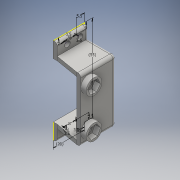
# Autodesk Inventor part: SwitchMount
Saved by Autodesk Inventor 2016 (Build 200138000, 138)
## iProperties
Created: 2026-04-02
Part Number: SwitchMount
Material: Generic
Document SubType Name: Modeling
Designer: Steve
Density: 1 g/cm^3
Appearance: Default
Author: Steve
Autodesk Inventor part; units mm, degrees
ref_plane "YZ Plane" through (0, 0, 0) normal (1, 0, 0) x (0, 1, 0)
ref_plane "XZ Plane" through (0, 0, 0) normal (0, 1, 0) x (-1, 0, 0)
ref_plane "XY Plane" through (0, 0, 0) normal (0, 0, 1) x (1, 0, 0)
sketch "Sketch1" plane through (0, 0, 0) normal (0, 1, 0) x (-1, 0, 0)
  line L0 (10, 17.5) -> (-10, 17.5)
  line L1 (-10, 17.5) -> (-10, -17.5)
  line L2 (-10, -17.5) -> (10, -17.5)
  line L3 (10, -17.5) -> (10, 17.5)
  line L4 (6.5, 5.2) -> (-6.5, 5.2)
  line L5 (-6.5, 5.2) -> (-6.5, -14)
  line L6 (-6.5, -14) -> (6.5, -14)
  line L7 (6.5, -14) -> (6.5, 5.2)
  circle A0 centre (5, 12.5) radius 2.55
  line L8 (7.6, 6.2) -> (-7.6, 6.2)
  line L9 (-7.6, 6.2) -> (-7.6, -15)
  line L10 (-7.6, -15) -> (7.6, -15)
  line L11 (7.6, -15) -> (7.6, 6.2)
  point P0 (0, 0)
  dimension "d0" = 35
  dimension "d1" = 20
  dimension "d2" = 17.5
  dimension "d3" = 10
  dimension "d4" = 19.2
  dimension "d5" = 13
  dimension "d6" = 3.5
  dimension "d7" = 3.5
  dimension "d8" = 5.1
  dimension "d9" = 5
  dimension "d10" = 5
  dimension "d11" = 1.1
  dimension "d12" = 1.1
  dimension "d13" = 15.2
  dimension "d14" = 1
  dimension "d15" = 1
  dimension "d16" = 21.2
  dimension "d42" = 6.3
  constraints: 24 end point, 6 parallel, 3 horizontal, 3 perpendicular, 1 centre point
  measures "d0" distance of L2.end L0.start
  measures "d1" distance of L1.end L2.end
  measures "d2" distance from line of L0 point (0, 0)
  measures "d3" distance from line of L3 point (0, 0)
  measures "d4" distance of L6.end L4.start
  measures "d5" distance of L5.end L6.end
  measures "d6" distance between parallel lines of L3 L7
  measures "d7" distance between parallel lines of L2 L6
  measures "d8" diameter of A0
  measures "d9" distance from line of L3 A0.centre
  measures "d10" distance from line of L0 A0.centre
  measures "d11" distance between parallel lines of L11 L7
  measures "d12" distance between parallel lines of L9 L5
  measures "d13" distance of L9.end L10.end
  measures "d14" distance between parallel lines of L8 L4
  measures "d15" distance between parallel lines of L10 L6
  measures "d16" distance of L10.end L8.start
  measures "d42" distance from line of L8 A0.centre
extrude "Extrusion1" add sketch "Sketch1" along normal blind 2.5 contours L3 L2 L1 L0
extrude "Extrusion2" add sketch "Sketch1" along normal blind 1.5 contours L11 L10 L9 L8
sketch "Sketch2" plane through (-10, 0, -17.5) normal (-1, 0, 0) x (0, 0, 1)
  line L0 (35, 2.5) -> (0, 2.5) projected
  line L1 (0, 2.5) -> (-10, 2.5)
  line L2 (-10, 2.5) -> (-10, -17.5)
  line L3 (-10, -17.5) -> (0, -17.5)
  line L4 (0, -17.5) -> (0, 2.5)
  line L5 (35, 2.5) -> (45, 2.5)
  line L6 (45, 2.5) -> (45, -17.5)
  line L7 (45, -17.5) -> (35, -17.5)
  line L8 (35, -17.5) -> (35, 2.5)
  point P0 (17.5, 0)
  dimension "d21" = 10
  dimension "d22" = 20
  dimension "d23" = 10
  dimension "d24" = 20
  constraints: 16 end point, 4 parallel, 2 horizontal, 2 perpendicular
  measures "d21" distance of L3.end L2.end
  measures "d22" distance of L2.end L1.end
  measures "d23" distance of L6.end L7.end
  measures "d24" distance of L5.end L6.end
extrude "Extrusion3" add sketch "Sketch2" against normal blind 2.5
sketch "Sketch3" plane through (-10, -17.5, -27.5) normal (-1, 0, 0) x (0, 0, 1)
  circle A0 centre (51, 14.5) radius 1.75
  circle A1 centre (4, 14.5) radius 1.75
  circle A2 centre (4, 6.5) radius 1.75
  line L0 (55, 20) -> (0, 20) projected
  line L1 (0, 0) -> (10, 0) projected
  line L2 (55, 0) -> (55, 20) projected
  line L3 (0, 20) -> (0, 0) projected
  circle A3 centre (51, 6.5) radius 1.75
  point P0 (27.5, 17.5)
  dimension "d27" = 3.5
  dimension "d28" = 3.5
  dimension "d29" = 3.5
  dimension "d30" = 5.5
  dimension "d31" = 5.5
  dimension "d32" = 8
  dimension "d34" = 4
  dimension "d35" = 4
  dimension "d36" = 4
  dimension "d83" = 3.5
  dimension "d84" = 4
  dimension "d85" = 8
  dimension "d113" = 20
  dimension "d114" = 55
  constraints: 4 centre point
  measures "d27" diameter of A0
  measures "d28" diameter of A1
  measures "d29" diameter of A2
  measures "d30" distance from line of L0 A0.centre
  measures "d31" distance from line of L0 A1.centre
  measures "d32" distance of A2.centre A1.centre
  measures "d34" distance from line of L2 A0.centre
  measures "d35" distance from line of L3 A1.centre
  measures "d36" distance from line of L3 A2.centre
  measures "d83" diameter of A3
  measures "d84" distance from line of L2 A3.centre
  measures "d85" distance of A0.centre A3.centre
  measures "d113" distance of L0.end L1.start
  measures "d114" distance of L0.start L0.end
sketch "Sketch5" plane through (0, 0, 0) normal (0, -1, 0) x (1, 0, 0)
  line L0 (10, 17.5) -> (10, -17.5) projected
  line L1 (-7.5, 17.5) -> (10, 17.5) projected
  line L2 (10, -17.5) -> (7.5, -17.5)
  line L3 (7.5, -17.5) -> (7.5, 17.5)
  line L4 (7.5, 17.5) -> (10, 17.5)
  line L5 (10, 17.5) -> (10, -17.5)
  point P0 (0, 0)
  dimension "d41" = 2.5
  constraints: 8 end point, 2 parallel, 1 horizontal, 1 perpendicular, 1 point on line
  measures "d41" distance of L3.end L4.end
extrude "Extrusion6" add sketch "Sketch5" along normal blind 20
sketch "Sketch9" plane through (-7.5, 2.5, 17.5) normal (0, 0, 1) x (1, 0, 0)
  line L0 (0, 0) -> (17.5, 0) projected
  line L1 (17.5, -22.5) -> (17.5, 0) projected
  line L2 (17.5, 0) -> (17.5, -22.5)
  line L3 (17.5, -22.5) -> (15, -22.5)
  line L4 (15, -22.5) -> (0, -20)
  line L5 (0, -20) -> (0, 0)
  line L6 (0, 0) -> (17.5, 0)
  point P0 (7.5, -2.5)
  constraints: 10 end point, 1 collinear, 1 parallel, 1 perpendicular, 1 vertical
extrude "Extrusion11" add sketch "Sketch9" along normal blind 2.5
sketch "Sketch11" plane through (10, 2.5, -17.5) normal (0, 0, -1) x (-1, 0, 0)
  line L0 (0, 0) -> (17.5, 0) projected
  line L1 (17.5, 0) -> (0, 0)
  line L2 (0, 0) -> (0, -22.5)
  line L3 (2.5, -22.5) -> (0, -22.5) projected
  line L4 (0, -22.5) -> (2.5, -22.5)
  line L5 (17.5, -20) -> (2.5, -22.5) projected
  line L6 (2.5, -22.5) -> (17.5, -20)
  line L7 (17.5, -20) -> (17.5, 0)
  point P0 (10, -2.5)
  constraints: 10 end point, 2 collinear, 1 horizontal, 1 parallel, 1 perpendicular
extrude "Extrusion12" add sketch "Sketch11" along normal blind 2.5
fillet "Fillet1" radius 2 11 edges at (-7.5, -7.5, 27.5) (-8.75, 2.5, 27.5) (-7.5, 2.5, 23.75) (-7.5, 2.5, -23.75) (-8.75, 2.5, -27.5) (-7.5, -7.5, -27.5) (1.25, 2.5, -20) (10, 2.5, 0) (1.25, 2.5, 20) (10, -8.75, 20) (10, -8.75, -20)
extrude "Extrusion15" cut sketch "Sketch3" against normal blind 10
extrude "Extrusion16" add sketch "Sketch1" along normal blind 2.5 contours L11 L10 L9 L8
chamfer "Chamfer2" distance 2 angle 45 2 edges at (0, 0, 5.2) (0, 0, -14)
sketch "Sketch14" plane through (7.5, 0, -17.5) normal (-1, 0, 0) x (0, 0, 1)
  circle A0 centre (5, -15) radius 2.25
  circle A1 centre (30, -15) radius 2.25
  line L0 (35, -20) -> (0, -20) projected
  line L1 (0, -17.5) -> (0, 0) projected
  line L2 (35, 0) -> (35, -17.5) projected
  circle A2 centre (5, -15) radius 5
  circle A3 centre (30, -15) radius 5
  point P0 (17.5, 0)
  dimension "d97" = 4.5
  dimension "d98" = 4.5
  dimension "d99" = 5
  dimension "d100" = 5
  dimension "d101" = 5
  dimension "d102" = 5
  dimension "d105" = 10
  dimension "d106" = 10
  constraints: 4 centre point, 2 coincident
  measures "d97" diameter of A1
  measures "d98" diameter of A0
  measures "d99" distance from line of L0 A0.centre
  measures "d100" distance from line of L1 A0.centre
  measures "d101" distance from line of A1.centre L0
  measures "d102" distance from line of L2 A1.centre
  measures "d105" diameter of A2
  measures "d106" diameter of A3
extrude "Extrusion17" cut sketch "Sketch14" against normal blind 2.5 contours A0 | A1
extrude "Extrusion18" add sketch "Sketch14" against normal blind 6
sketch "Sketch15" plane through (13.5, -15, -12.5) normal (1, 0, 0) x (0, 0, -1)
  line L0 (-3.6792, 1.8074) -> (-0.2743, 4.09)
  line L1 (-0.2743, 4.09) -> (3.4049, 2.2826)
  line L2 (3.4049, 2.2826) -> (3.6792, -1.8074)
  line L3 (3.6792, -1.8074) -> (0.2743, -4.09)
  line L4 (0.2743, -4.09) -> (-3.4049, -2.2826)
  line L5 (-3.4049, -2.2826) -> (-3.6792, 1.8074)
  line L6 (-28.2597, 2.4152) -> (-24.512, 4.076)
  line L7 (-24.512, 4.076) -> (-21.1999, 1.6608)
  line L8 (-21.1999, 1.6608) -> (-21.6355, -2.4152)
  line L9 (-21.6355, -2.4152) -> (-25.3831, -4.076)
  line L10 (-25.3831, -4.076) -> (-28.6953, -1.6608)
  line L11 (-28.6953, -1.6608) -> (-28.2597, 2.4152)
  point P0 (-12.5, 15)
  point P1 (0, 0)
  point P2 (-24.9476, 0)
  dimension "d109" = 7.1
  dimension "d110" = 7.1
  constraints: 24 end point, 26 other
  measures "d109" distance between parallel lines of L4 L1
  measures "d110" distance between parallel lines of L10 L7
extrude "Extrusion19" cut sketch "Sketch15" against normal blind 3.5
body "Solid1"
